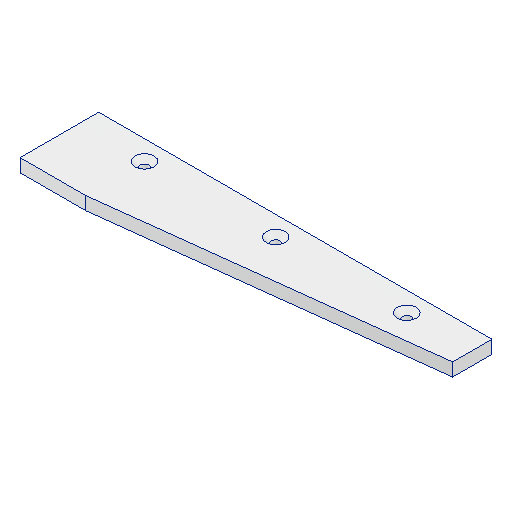
# Autodesk Inventor part: Chapa Suporte 2L (Trilho Roletado)
Saved by Autodesk Inventor 2026.1 (Build 301233000, 233)
## iProperties
Company: Elgin
Created: 2025-09-16
Part Number: Chapa Suporte 2L (Trilho Roletado)
Checked By: Antonio Lucas
Engr Approved By: Antonio Lucas
Material: Aluminio 1060
Document SubType Name: Modeling
Mfg Approved By: Anderson Oliveira
Designer: Willian Pinheiro
Mass: 378.716 g
Surface Area: 362.743 cm^2
Volume: 140.265 cm^3
Density: 2.7 g/cm^3
Appearance: Alumínio - Plano
Description: Chapa Suporte 2L (Trilho Roletado)
Dimensões: 10 x 60 x 300 mm
Total: 2
Author: Willian Pinheiro
Title: Ceteva
Revision Number: 00
Autodesk Inventor part; units mm, degrees
ref_plane "YZ Plane" through (0, 0, 0) normal (1, 0, 0) x (0, 1, 0)
ref_plane "XZ Plane" through (0, 0, 0) normal (0, 1, 0) x (-1, 0, 0)
ref_plane "XY Plane" through (0, 0, 0) normal (0, 0, 1) x (1, 0, 0)
sketch "Esboço1" plane through (0, 0, 0) normal (0, 0, 1) x (1, 0, 0)
  line L0 (-210, 0) -> (210, 0) construction
  line L1 (0, -42) -> (0, 42) construction
  line L2 (-150, 30) -> (150, 30)
  line L3 (150, 30) -> (150, -30)
  line L4 (150, -30) -> (-150, -30)
  line L5 (-150, -30) -> (-150, 30)
  line L6 (-150, 15) -> (150, 15) construction
  line L7 (-150, -15) -> (150, -15) construction
  line L8 (-150, 0) -> (100, -30)
  point P0 (0, 0)
  point P1 (-100, 15)
  point P2 (-100, -15)
  point P3 (100, 15)
  point P4 (100, -15)
  point P5 (0, 15)
  point P6 (0, -15)
  dimension "d0" = 60
  dimension "d1" = 300
  dimension "d2" = 30
  dimension "d3" = 100
  dimension "d24" = 250
  constraints: 14 end point, 7 point on line, 4 symmetric about line, 3 midpoint, 2 parallel, 2 perpendicular, 1 horizontal, 1 vertical alignment, 2 other
  measures "d0" distance between parallel lines of L4 L2
  measures "d1" distance of L2.start L2.end
  measures "d2" distance between parallel lines of L7 L6
  measures "d3" distance of point (0, 15) point (-100, 15)
  measures "d24" horizontal distance of L8.start L8.end
extrude "Extrusão1" add sketch "Esboço1" along normal mid plane 10 contours L2 L3 L4 L8 L5
sketch "Esboço2" plane through (0, 0, 5) normal (0, 0, 1) x (1, 0, 0)
  point P0 (0, 0)
  point P1 (-100, 15)
  point P2 (-100, -15)
  point P3 (0, 15)
  point P4 (0, -15)
  point P5 (100, 15)
  point P6 (100, -15)
hole "Furo1" at (-100, 15, 5) at (0, 15, 5) at (100, 15, 5) direction (0, 0, -1) diameter 6.5 end through all countersink diameter 14.5 countersink angle 90 clearance for "Countersunk Flat Head Hex Socket Screw ISO 10642" size "M6" standard "ISO"
sketch "Esboço3" plane through (150, -30, 5) normal (1, 0, 0) x (0, 0, -1)
  line L0 (12, 30) -> (-2, 30) construction
  line L1 (5, -12) -> (5, 72) construction
  point P0 (5, 30)
  point P1 (5, 45)
  point P2 (5, 15)
  dimension "d16" = 30
  constraints: 2 point on line, 1 symmetric about line
  measures "d16" distance of point (5, 15) point (5, 45)
hole "Furo2" at (150, 15, 0) at (150, -15, 0) direction (-1, 0, 0) diameter 4.134 depth 20 tip angle 118 thread size "M5x0.8" class "6H" standard "ISO Metric profile"
mirror "Espelhar1" about plane through (0, 0, 0) normal (1, 0, 0) remove original yes
